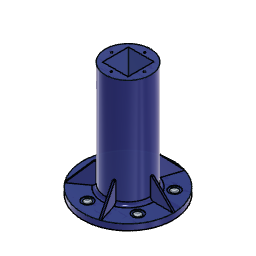
Base robótica 3.0 v12 (Autodesk Fusion 360 design; units mm, degrees)
Autodesk Fusion 360 part; units mm, degrees
sketch "Sketch1" plane through (0, 0, 0) normal (0, 0, 1) x (1, 0, 0)
  circle A0 centre (0, 0) radius 75
  dimension "d1" = 150
  constraint coincident A0.centre origin
  measures "d1" diameter of A0
extrude "Extrude1" add sketch "Sketch1" along normal blind 10 makes body 1
sketch "Sketch2" plane through (0, 0, 10) normal (0, 0, 1) x (-1, 0, 0)
  circle A0 centre (0, 0) radius 75
sketch "Sketch3" plane through (0, 0, 10) normal (0, 0, 1) x (-1, 0, 0)
  circle A0 centre (0, 0) radius 37.5
  dimension "d4" = 75
  constraint coincident A0.centre origin
  measures "d4" diameter of A0
extrude "Extrude2" add sketch "Sketch3" along normal blind 200 bodies 1
sketch "Sketch4" plane through (0, 0, 10) normal (0, 0, 1) x (-1, 0, 0)
  circle A0 centre (0, 0) radius 37.5
  line L0 (60.6763, 44.0839) -> (28.3156, 20.5725)
  line L1 (-23.1763, 71.3292) -> (-10.8156, 33.287)
  line L2 (-75, 0) -> (-35, 0)
  line L3 (-23.1763, -71.3292) -> (-10.8156, -33.287)
  line L4 (60.6763, -44.0839) -> (28.3156, -20.5725)
  line L5 (75, 0) -> (55, 0)
  line L6 (75, 0) -> (55, 0)
  line L7 (23.1763, 71.3292) -> (16.9959, 52.3081)
  line L8 (-60.6763, 44.0839) -> (-44.4959, 32.3282)
  line L9 (-60.6763, -44.0839) -> (-44.4959, -32.3282)
  line L10 (23.1763, -71.3292) -> (16.9959, -52.3081)
  line L11 (-10.8156, 33.287) -> (-23.1763, 71.3292)
  line L12 (-23.1763, 71.3292) -> (-26.0294, 70.4022)
  line L13 (-26.0294, 70.4022) -> (-13.6688, 32.3599)
  line L14 (-13.6688, 32.3599) -> (-10.8156, 33.287)
  line L15 (-75, 0) -> (-75, -3)
  line L16 (-35, -3) -> (-35, 0)
  line L17 (-75, -3) -> (-35, -3)
  line L18 (-23.1763, -71.3292) -> (-20.3231, -72.2563)
  line L19 (-7.9624, -34.214) -> (-10.8156, -33.287)
  line L20 (-20.3231, -72.2563) -> (-7.9624, -34.214)
  line L21 (60.6763, -44.0839) -> (62.4396, -41.6568)
  line L22 (30.079, -18.1454) -> (28.3156, -20.5725)
  line L23 (62.4396, -41.6568) -> (30.079, -18.1454)
  line L24 (60.6763, 44.0839) -> (58.9129, 46.5109)
  line L25 (26.5522, 22.9995) -> (28.3156, 20.5725)
  line L26 (58.9129, 46.5109) -> (26.5522, 22.9995)
  point P0 (75, 0)
  dimension "d9" = 20
  dimension "d11" = 360
  dimension "d12" = 3
  dimension "d14" = 360
  constraint coincident P0 L5.start
  constraint parallel L5 L6
  constraint perpendicular L11 L12
  constraint parallel L11 L13
  constraint parallel L12 L14
  measures "d9" distance of P0 L5.end
  measures "d12" distance of L1.end L13.end
extrude "Extrude3" add sketch "Sketch4" along normal blind 35 separate body contours A0 L0 L25 L26 | A0 L0 L24 L26 | A0 L4 L21 L23 | A0 L4 L22 L23 | A0 L1 L11 L13 L14 | A0 L1 L11 L12 L13 | A0 L3 L18 L20 | A0 L3 L19 L20 | A0 L2 L16 L17 | A0 L2 L15 L17 makes body 2 at (16.2029, 59.5755, 21.6667) makes body 3 at (19.056, -58.6485, 33.3333) makes body 4 at (-48.126, -38.6738, 33.3333) makes body 5 at (61.6667, 3, 33.3333) makes body 6 at (-49.8894, 36.2468, 33.3333)
sketch "Sketch5" plane through (0, 0, 10) normal (0, 0, 1) x (-1, 0, 0)
  line L0 (75, 3) -> (55, 3)
  line L1 (20.3231, 72.2563) -> (14.1428, 53.2352)
  line L2 (-62.4396, 41.6568) -> (-46.2593, 29.9011)
  line L3 (-58.9129, -46.5109) -> (-42.7326, -34.7552)
  line L4 (26.0294, -70.4022) -> (19.8491, -51.3811)
  point P0 (62.4396, -41.6568)
  point P1 (30.079, -18.1454)
  dimension "d19" = 20
  dimension "d21" = 360
  measures "d19" distance of L0.start L0.end
hole "Hole1" at (-55, -3, 10) at (-14.1428, -53.2352, 10) at (-19.8491, 51.3811, 10) at (42.7326, 34.7552, 10) at (46.2593, -29.9011, 10) direction (0, 0, -1) diameter 12.023 depth 10 tip angle 118 counterbore diameter 18 counterbore depth 1 bodies 1
thread "Thread1" "ISO Metric profile 14.0 M14x2 6H"
fillet "Fillet1" radius 5 1 edges at (34.9623, -13.5606, 10) on bodies 1
combine "Combine1" operation add target body 1 tool bodies 4 3 5 6 2
chamfer "Chamfer1" distance 35 distance2 35 5 edges at (75, 1.5, 45) (21.7497, 71.7928, 45) (-61.558, 42.8704, 45) (24.6029, -70.8657, 45) (-59.7946, -45.2974, 45) measured on face at (62.4955, 1.3337, 45) measured on face at (18.0438, 59.8489, 45) measured on face at (-51.3439, 35.655, 45) measured on face at (20.5806, -59.0247, 45) measured on face at (-49.7761, -37.8129, 45) on bodies 1
sketch "Sketch6" plane through (0, 0, 210) normal (0, 0, 1) x (-1, 0, 0)
  circle A0 centre (0, 0) radius 37.5
  line L0 (-21.209, 21.209) -> (21.209, 21.209)
  line L1 (21.209, 21.209) -> (21.209, -21.209)
  line L2 (21.209, -21.209) -> (-21.209, -21.209)
  line L3 (-21.209, -21.209) -> (-21.209, 21.209)
  line L4 (-21.209, 21.209) -> (21.209, -21.209) construction
  line L5 (21.209, 21.209) -> (-21.209, -21.209) construction
  dimension "d31" = 42.418
  dimension "d32" = 42.418
  constraint horizontal L0
  constraint perpendicular L0 L1
  constraint parallel L0 L2
  constraint parallel L1 L3
  constraint coincident L4 A0.centre
  constraint coincident L5 A0.centre
  constraint coincident A0.centre origin
  measures "d31" distance of L1.end L2.end
  measures "d32" distance of L0.end L1.end
extrude "Extrude9" cut 1 faces at (-9.3028, -10.3652, 210) along direction (0, 0, -1) blind 20 on bodies 1 bodies 1
sketch "Sketch22" plane through (0, 0, 190) normal (0, 0, 1) x (-1, 0, 0)
  circle A0 centre (0, 0) radius 37.5
sketch "Sketch23" plane through (0, 0, 190) normal (0, 0, 1) x (-1, 0, 0)
  line L0 (-21.2, -21.2) -> (21.2, -21.2)
  line L1 (21.2, -21.2) -> (21.2, 21.2)
  line L2 (21.2, 21.2) -> (-21.2, 21.2)
  line L3 (-21.2, 21.2) -> (-21.2, -21.2)
  line L4 (-21.2, -21.2) -> (21.2, 21.2) construction
  line L5 (21.2, -21.2) -> (-21.2, 21.2) construction
  dimension "d103" = 42.4
  dimension "d104" = 42.4
  constraint horizontal L0
  constraint perpendicular L0 L1
  constraint parallel L0 L2
  constraint parallel L1 L3
  constraint coincident L4 origin
  constraint coincident L5 origin
  measures "d103" distance of L1.end L2.end
  measures "d104" distance of L0.end L1.end
extrude "Extrude10" cut sketch "Sketch23" against normal blind 48.006 bodies 1
sketch "Sketch24" plane through (0, 0, 190) normal (0, 0, 1) x (-1, 0, 0)
  line L0 (21.2, -21.2) -> (21.2, -21.962)
  line L1 (-21.2, -21.2) -> (-21.2, -21.962)
  line L2 (21.2, -21.2) -> (-21.2, -21.2)
  line L3 (-21.2, -21.962) -> (21.2, -21.962)
  point P0 (21.2, -21.2)
  point P1 (-21.2, -21.2)
  dimension "d107" = 0.762
  dimension "d108" = 0.762
  constraint coincident P0 L0.start
  constraint vertical L0
  constraint coincident P1 L1.start
  constraint vertical L1
  measures "d107" distance of P0 L0.end
  measures "d108" distance of P1 L1.end
extrude "Extrude11" cut sketch "Sketch24" against normal blind 48.006 bodies 1
sketch "Sketch26" plane through (0, 21.962, 0) normal (0, -1, 0) x (1, 0, 0)
  line L0 (21.2, 190) -> (-21.2, 190)
  line L1 (-21.2, 190) -> (-21.2, 141.994)
  line L2 (-21.2, 141.994) -> (21.2, 141.994)
  line L3 (21.2, 141.994) -> (21.2, 190)
  line L4 (0, 141.994) -> (0, 142.248)
  line L5 (0, 142.248) -> (5.715, 142.248)
  line L6 (0, 142.248) -> (-5.715, 142.248)
  line L7 (5.715, 142.248) -> (5.715, 151.341)
  line L8 (-5.715, 142.248) -> (-5.715, 151.341)
  line L9 (-5.715, 151.341) -> (5.715, 151.341)
  dimension "d111" = 0.254
  dimension "d112" = 5.715
  dimension "d113" = 5.715
  dimension "d114" = 9.093
  dimension "d115" = 9.093
  constraint midpoint L2 L4.start
  constraint vertical L4
  constraint perpendicular L4 L5
  constraint perpendicular L4 L6
  constraint perpendicular L2 L7
  constraint perpendicular L6 L8
  measures "d111" distance of L4.start L4.end
  measures "d112" distance of L4.end L5.end
  measures "d113" distance of L4.end L6.end
  measures "d114" distance of L5.end L7.end
  measures "d115" distance of L6.end L8.end
extrude "Extrude12" cut sketch "Sketch26" against normal blind 55 contours L5 L6 L7 L8 L9 bodies 1
sketch "Sketch27" plane through (0, 0, 190) normal (0, 0, 1) x (-1, 0, 0)
  circle A0 centre (0, 0) radius 37.5
  line L0 (-0.1682, -37.4996) -> (-0.1233, -27.4997)
  line L1 (37.4996, -0.1682) -> (27.4997, -0.1233)
  line L2 (0.1682, 37.4996) -> (0.1233, 27.4997)
  line L3 (-37.4996, 0.1682) -> (-27.4997, 0.1233)
  dimension "d118" = 10
  dimension "d120" = 360
  constraint coincident A0 L0.start
  measures "d118" distance of L0.start L0.end
hole "Hole5" at (27.4997, -0.1233, 190) at (-0.1233, -27.4997, 190) at (0.1233, 27.4997, 190) at (-27.4997, 0.1233, 190) direction (0, 0, -1) diameter 3.332 depth 35 tip angle 118 bodies 1
thread "Thread5" "ISO Metric profile 4.0 M4x0.7 6H"
